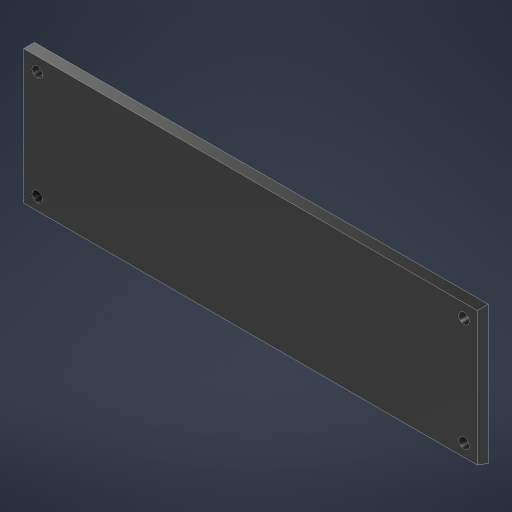
# Autodesk Inventor part: góra_robota
Saved by Autodesk Inventor 2023.4 (Build 274418000, 418)
## iProperties
Created: 2025-10-31
Part Number: góra_robota
Material: Tworzywo sztuczne PET
Document SubType Name: Modeling
Designer: Jakub Borsukiewicz
Density: 1.541 g/cm^3
Appearance: Lśniąca — czarna
Author: Jakub Borsukiewicz
Autodesk Inventor part; units mm, degrees
ref_plane "YZ Plane" through (0, 0, 0) normal (1, 0, 0) x (0, 1, 0)
ref_plane "XZ Plane" through (0, 0, 0) normal (0, 1, 0) x (-1, 0, 0)
ref_plane "XY Plane" through (0, 0, 0) normal (0, 0, 1) x (1, 0, 0)
sketch "Szkic1" plane through (0, 0, 0) normal (0, 0, 1) x (1, 0, 0)
  line L0 (-8.4, 0) -> (50.4, 0) projected
  line L1 (0, -5.1) -> (0, 30.6) projected
  line L2 (0, 0) -> (42, 0)
  line L3 (42, 0) -> (42, 25.5)
  line L4 (42, 25.5) -> (0, 25.5)
  line L5 (0, 25.5) -> (0, 0)
  circle A0 centre (39.5, 23) radius 1
  circle A1 centre (39.5, 3) radius 1
  point P0 (0, 25.5)
  point P1 (42, 0)
  dimension "d0" = 25.5
  dimension "d1" = 42
  dimension "d7" = 2
  dimension "d8" = 2
  dimension "d9" = 2.5
  dimension "d10" = 2.5
  dimension "d11" = 20
  dimension "d12" = 2.5
  constraints: 8 end point, 2 centre point, 2 parallel, 1 horizontal, 1 perpendicular
  measures "d0" distance of L2.end L3.end
  measures "d1" distance of L3.end L4.end
  measures "d7" diameter of A0
  measures "d8" diameter of A1
  measures "d9" distance from line of L4 A0.centre
  measures "d10" distance from line of L3 A0.centre
  measures "d11" distance of A1.centre A0.centre
  measures "d12" distance from line of L3 A1.centre
extrude "Wyciągnięcie proste1" add sketch "Szkic1" along normal blind 2
sketch "Szkic2" plane through (42, 0, 0) normal (1, 0, 0) x (0, 0, -1)
  line L0 (0, 0) -> (0, 25.5) projected
  line L1 (0, 25.5) -> (-2, 25.5) projected
  line L2 (-2, 0) -> (-2, 25.5) projected
  line L3 (0, 0) -> (-2, 0) projected
  line L4 (0, 25.5) -> (0, 0) projected
  line L5 (0, 0) -> (-2, 0.7279)
  line L6 (-2, 25.5) -> (-2, 0) projected
  point P0 (0, 0)
  dimension "d4" = 70
  constraints: 2 end point, 1 point on line
  measures "d4" angle of L0 L5
extrude "Wyciągnięcie proste2" cut sketch "Szkic2" against normal blind 90 contours L3 L2 L5
mirror "Odbij1" about plane through (0, 0, 0) normal (1, 0, 0) of "Wyciągnięcie proste1", "Wyciągnięcie proste2"
